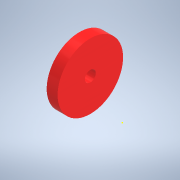
# Autodesk Inventor part: clutch02-simplyGearDisk
Saved by Autodesk Inventor 2021 (Build 250183000, 183)
## iProperties
Created: 2020-07-03
Part Number: clutch02-simplyGearDisk
Material: PET Plastic
Document SubType Name: Modeling
Designer: robst
Density: 1.541 g/cm^3
Appearance: Light Red
Author: robst
Autodesk Inventor part; units mm, degrees
ref_plane "YZ Plane" through (0, 0, 0) normal (1, 0, 0) x (0, 1, 0)
ref_plane "XZ Plane" through (0, 0, 0) normal (0, 1, 0) x (-1, 0, 0)
ref_plane "XY Plane" through (0, 0, 0) normal (0, 0, 1) x (1, 0, 0)
ref_plane "Work Plane1" through (-110.2685, -72.0125, 201.5707) normal (-1, 0, 0) x (0, -1, 0)
sketch "Sketch1" plane through (-110.2685, -72.0125, 201.5707) normal (-1, 0, 0) x (0, -1, 0)
  circle A0 centre (-228.6, -101.6) radius 12.7 projected
  circle A1 centre (-228.6, -101.6) radius 76.2
  circle A2 centre (-228.6, -101.6) radius 12.7
  point P0 (-72.0125, -201.5707)
  dimension "d0" = 152.4
  constraints: 2 centre point, 2 coincident, 1 concentric
  measures "d0" diameter of A1
extrude "Extrusion1" add sketch "Sketch1" along normal blind 25.4
sketch "Sketch2" plane through (-135.6685, 156.5875, 99.9707) normal (-1, 0, 0) x (0, 0, 1)
  point P0 (-99.9707, -156.5875)
body "Solid1"
